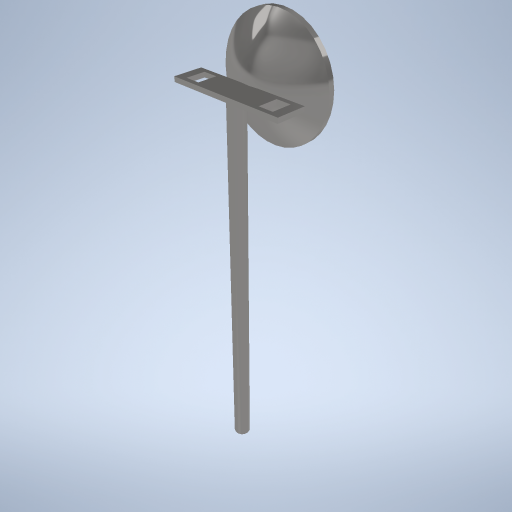
# Autodesk Inventor part: hubble_antenna
Saved by Autodesk Inventor 2024 (Build 280153000, 153)
## iProperties
Created: 2024-04-16
Part Number: hubble_antenna
Material: Stainless Steel AISI 440C, Welded
Document SubType Name: Modeling
Designer: soham
Density: 7.8 g/cm^3
Appearance: Steel - Polished
Author: soham
Autodesk Inventor part; units mm, degrees
ref_plane "YZ Plane" through (0, 0, 0) normal (1, 0, 0) x (0, 1, 0)
sketch "pole_sketch" plane through (0, 0, 0) normal (0, 0, 1) x (1, 0, 0)
  line L0 (0, 0) -> (0, 480)
  line L1 (-8.65, 0) -> (-8.65, 400)
  line L2 (-8.65, 0) -> (0, 0)
  line L3 (-8.65, 400) -> (0, 400)
  dimension "d0" = 480
  dimension "d1" = 17.3
  dimension "d2" = 400
  constraints: 8 end point, 2 vertical, 1 horizontal, 1 perpendicular, 1 point on line
  measures "d0" distance of L0.start L0.end
  measures "d1" diameter of L1 L0
  measures "d2" distance of L1.start L1.end
revolve "pole_revolve" add sketch "pole_sketch" angle 360 about axis through (0, 0, 0) along (0, 1, 0)
ref_plane "Work Plane1" through (0, 400, 0) normal (0, 1, 0) x (-1, 0, 0)
sketch "dish_support_sketch" plane through (0, 400, 0) normal (0, 1, 0) x (-1, 0, 0)
  line L0 (60, -15) -> (60, 15)
  line L1 (60, 15) -> (-60, 15)
  line L2 (-60, 15) -> (-60, -15)
  line L3 (-60, -15) -> (60, -15)
  line L4 (-84, 0) -> (84, 0) projected
  line L5 (0, -21) -> (0, 21) projected
  line L6 (50, -10) -> (50, 10)
  line L7 (50, 10) -> (35, 10)
  line L8 (35, 10) -> (35, -10)
  line L9 (35, -10) -> (50, -10)
  line L10 (-50, -10) -> (-50, 10)
  line L11 (-50, 10) -> (-35, 10)
  line L12 (-35, 10) -> (-35, -10)
  line L13 (-35, -10) -> (-50, -10)
  point P0 (0, 0)
  dimension "d6" = 30
  dimension "d7" = 15
  dimension "d8" = 120
  dimension "d9" = 60
  dimension "d10" = 10
  dimension "d11" = 15
  dimension "d12" = 20
  dimension "d13" = 10
  constraints: 24 end point, 7 perpendicular, 4 symmetric about line, 1 vertical
  measures "d6" distance of L0.start L0.end
  measures "d7" distance between parallel lines of L3 L4
  measures "d8" distance between parallel lines of L2 L0
  measures "d9" distance between parallel lines of L5 L0
  measures "d10" distance between parallel lines of L6 L0
  measures "d11" distance of L8.end L6.start
  measures "d12" distance of L7.end L8.end
  measures "d13" distance between parallel lines of L4 L9
extrude "dish_support_extrude" add sketch "dish_support_sketch" along normal blind 5 contours L3 L5 L4 L8 L9 L6 L0 | L4 L6 L7 L8 L5 L1 L0 | L3 L2 L4 L10 L13 L12 L5 | L4 L12 L11 L10 L2 L1 L5
ref_plane "Work Plane2" through (0, 402.5, 0) normal (0, 1, 0) x (-1, 0, 0)
sketch "dish_sketch" plane through (0, 402.5, 0) normal (0, 1, 0) x (-1, 0, 0)
  line L0 (60, 15) -> (-60, 15) projected
  line L1 (-60, -15) -> (60, -15) projected
  spline S0 degree 5 poles (0, -14) (6.2404, -14.0001) (12.4863, -14.811) (18.576, -16.4375) (31.4677, -21.4497) (43.0955, -28.9943) (49.0504, -33.6443) (54.6746, -38.6737) (60, -44) knots 0 0 0 0 0 0 0.453143 0.453143 0.453143 1 1 1 1 1 1
  line L2 (0, 0) -> (0, -150)
  line L3 (60, -50) -> (60, -44)
  spline S1 degree 5 poles (0, -30) (12.8337, -29.9985) (25.6927, -32.2934) (37.916, -36.8682) (49.316, -42.8763) (60, -50) knots 0 0 0 0 0 0 1 1 1 1 1 1
  point P0 (0, -15)
  dimension "d47" = 35
  dimension "d49" = 6
  dimension "d50" = 120
  dimension "d51" = 60
  dimension "d53" = 30
  dimension "d60" = 150
  constraints: 5 end point, 2 vertical, 1 midpoint, 6 other
  measures "d47" distance from line of L1 L3.start
  measures "d49" distance of L3.start L3.end
  measures "d50" diameter of L3.start L2
  measures "d51" horizontal distance of point (0, -30) L3.start
  measures "d53" vertical distance of point (0, -14) L3.end
  measures "d60" distance of L2.start L2.end
revolve "dish_revolve" add sketch "dish_sketch" angle 360 about axis through (0, 402.5, 0) along (0, 0, -1)
ref_plane "Work Plane4" through (0, 0, -30) normal (0, 0, 1) x (1, 0, 0)
sketch "interior_antenna_sketch" plane through (0, 402.5, 0) normal (0, 1, 0) x (-1, 0, 0)
  line L0 (-60, -50) -> (60, -50) projected
  line L1 (-84.4225, -30) -> (86.5349, -30) projected
  line L2 (0, -30) -> (0, -130)
  line L3 (2.5, -30.0347) -> (2.5, -50.0347)
  arc A0 (2.5, -30.0347) -> (0, -30) centre (-0.0058, -120.434) ccw
  arc A1 (0, -59.3648) -> (2.5, -50.0347) centre (0, -54.3648) ccw
  point P0 (0, 0)
  dimension "d38" = 20
  dimension "d39" = 5
  dimension "d40" = 90.434
  dimension "d41" = 5
  dimension "d61" = 100
  constraints: 4 end point, 4 point on circle, 2 centre point, 2 point on line, 2 vertical, 2 other
  measures "d38" distance of L3.start L3.end
  measures "d39" diameter of L3.end L2
  measures "d40" radius of A0
  measures "d41" radius of A1
  measures "d61" distance of L2.start L2.end
revolve "interior_antenna_revolve" add sketch "interior_antenna_sketch" angle 360 about axis through (0, 402.5, -30) along (0, 0, -1)
sketch "slot_sketch" plane through (0, 0, 0) normal (0, -1, 0) x (1, 0, 0)
  circle A0 centre (0, 0) radius 7.15
  dimension "d43" = 14.3
  constraints: 1 centre point, 1 coincident
  measures "d43" diameter of A0
extrude "slot_extrude" cut sketch "slot_sketch" against normal blind 133.3333
equation "\"d1\" = pole_diameter"
equation "\"d2\" = pole_height"
equation "\"d6\" = 0.25 * dish_width"
equation "\"d7\" = 0.125 * dish_width"
equation "\"d8\" = dish_width"
equation "\"d9\" = 0.5 * dish_width"
equation "\"d44\" = 0.333333 * pole_height"
equation "\"pole_diameter\" = 17.3"
equation "\"pole_height\" = 400"
equation "\"dish_width\" = 120"
equation "curve S0 of \"dish_sketch\": x = 6*t; y = -0.3*t^2 - dish_width/8+1; t from d17 to d18"
equation "curve S1 of \"dish_sketch\": x = 6*t; y = -0.2*t^2-30; t from d26 to d27"
body "Solid1"
